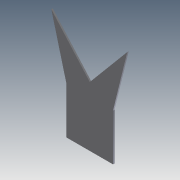
# Autodesk Inventor part: 130 view
Saved by Autodesk Inventor 2011 (Build 150239000, 239)
## iProperties
Created: 2012-01-08
Part Number: 130 view
Document SubType Name: Modeling
Designer: Matthew
Density: 1 g/cm^3
Author: Matthew
Autodesk Inventor part; units mm, degrees
ref_plane "YZ Plane" through (0, 0, 0) normal (1, 0, 0) x (0, 1, 0)
ref_plane "XZ Plane" through (0, 0, 0) normal (0, 1, 0) x (-1, 0, 0)
ref_plane "XY Plane" through (0, 0, 0) normal (0, 0, 1) x (1, 0, 0)
sketch "Sketch1" plane through (0, 0, 0) normal (0, 0, 1) x (1, 0, 0)
  line L0 (-16.301, -16.2161) -> (85.299, -16.2161)
  line L1 (85.299, -16.2161) -> (85.299, 85.3839)
  line L2 (85.299, 85.3839) -> (-16.301, 85.3839)
  line L3 (-16.301, 85.3839) -> (-16.301, -16.2161)
  line L4 (34.499, 85.3839) -> (34.499, -16.2161)
  line L5 (34.499, 34.5839) -> (66.7382, 61.6358)
  line L6 (34.499, 34.5839) -> (76.5843, 34.5839) construction
  line L7 (66.7382, 61.6358) -> (85.299, 77.2102)
  line L8 (34.499, 34.5839) -> (-7.0205, 69.423)
  line L9 (34.499, 34.5839) -> (88.699, 34.5839) construction
  line L10 (-7.0205, 69.423) -> (-16.301, 77.2102)
  line L11 (34.499, 34.5839) -> (-4.416, 67.2375)
  line L12 (-4.416, 67.2375) -> (-16.301, 53.0736)
  line L13 (-4.416, 67.2375) -> (10.8106, 85.3839)
  line L14 (34.499, 34.5839) -> (73.4141, 67.2375)
  line L15 (73.4141, 67.2375) -> (37.5423, 109.9879)
  line L16 (37.5423, 109.9879) -> (34.499, 113.6147)
  line L17 (10.8106, 85.3839) -> (34.499, 113.6147)
  line L18 (34.499, 113.6147) -> (-49.1377, 209.1861)
  line L19 (34.499, 113.6147) -> (116.1331, 210.9023)
  line L20 (116.1331, 210.9023) -> (85.299, 85.3839)
  line L21 (-16.301, 85.3839) -> (-49.1377, 209.1861)
  point P0 (0, 0)
  dimension "d0" = 101.6
  dimension "d1" = 101.6
  dimension "d2" = 40
  dimension "d3" = 140
  dimension "d4" = 50.8
  dimension "d5" = 50.8
  dimension "d6" = 127
  dimension "d7" = 127
  constraints: 44 end point, 6 collinear, 6 point on line, 3 horizontal, 3 midpoint, 3 perpendicular, 2 equal length, 2 parallel
  measures "d0" distance of L2.end L1.end
  measures "d1" distance of L1.end L0.end
  measures "d2" angle of L6 L5
  measures "d3" angle of L9 L8
  measures "d4" distance of L5.start L11.end
  measures "d5" distance of L5.start L14.end
  measures "d6" distance of L16.end L18.end
  measures "d7" distance of L16.end L19.end
extrude "Extrusion1" add sketch "Sketch1" along normal blind 3.175
body "Solid1"
